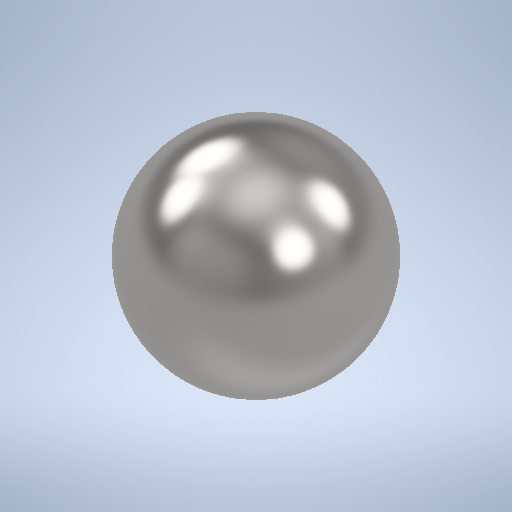
# Autodesk Inventor part: Gelenke
Saved by Autodesk Inventor 2025.2 (Build 292293000, 293)
## iProperties
Created: 2025-05-16
Part Number: Gelenke
Material: Steel, Alloy
Document SubType Name: Modeling
Designer: MSIGAMING
Mass: 32379.3 g
Surface Area: 1256.64 cm^2
Volume: 4188.79 cm^3
Density: 7.73 g/cm^3
Appearance: Semi-Polished
Author: MSIGAMING
Autodesk Inventor part; units mm, degrees
ref_plane "YZ Plane" through (0, 0, 0) normal (1, 0, 0) x (0, 1, 0)
ref_plane "XZ Plane" through (0, 0, 0) normal (0, 1, 0) x (-1, 0, 0)
ref_plane "XY Plane" through (0, 0, 0) normal (0, 0, 1) x (1, 0, 0)
sketch "Sketch1" plane through (0, 0, 0) normal (0, 1, 0) x (-1, 0, 0)
  arc A0 (100, 0) -> (-100, 0) centre (0, 0) ccw
  line L0 (-100, 0) -> (100, 0)
  arc A1 (95, 0) -> (-95, 0) centre (0, 0) ccw
  dimension "d0" = 200
  dimension "d2" = 190
  constraints: 4 point on circle, 2 centre point, 2 coincident, 2 end point, 2 point on line
  measures "d0" diameter of A0
  measures "d2" diameter of A1
revolve "Revolution1" add sketch "Sketch1" angle 360 about axis through (100, 0, 0) along (-1, 0, 0) contours L0 A1 A0
body "Solid1"
